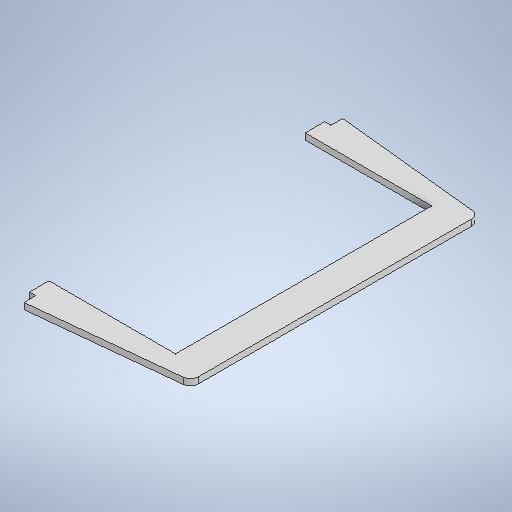
# Autodesk Inventor part: horazontal battery suport
Saved by Autodesk Inventor 2025.2 (Build 292293000, 293)
## iProperties
Created: 2025-01-25
Part Number: horazontal battery suport
Material: Generic
Document SubType Name: Modeling
Designer: alex
Density: 1 g/cm^3
Appearance: Default
Author: alex
Autodesk Inventor part; units mm, degrees
ref_plane "YZ Plane" through (0, 0, 0) normal (1, 0, 0) x (0, 1, 0)
ref_plane "XZ Plane" through (0, 0, 0) normal (0, 1, 0) x (-1, 0, 0)
ref_plane "XY Plane" through (0, 0, 0) normal (0, 0, 1) x (1, 0, 0)
sketch "Sketch1" plane through (0, 0, 0) normal (0, 1, 0) x (-1, 0, 0)
  line L0 (0, 0) -> (0, 31.75)
  line L1 (0, 31.75) -> (-10.16, 31.75)
  line L2 (-10.16, 31.75) -> (-10.16, 50.8)
  line L3 (-256.504, 13.9421) -> (-256.504, -430.5021)
  line L4 (-10.16, -467.36) -> (-10.16, -448.31)
  line L5 (-10.16, -448.31) -> (0, -448.31)
  line L6 (0, -448.31) -> (0, -416.56)
  line L7 (0, 0) -> (-205.704, 0)
  line L8 (-205.704, 0) -> (-205.704, -416.56)
  line L9 (-205.704, -416.56) -> (0, -416.56)
  line L10 (-245.1066, -443.1352) -> (-10.16, -467.36)
  line L11 (-245.1066, 26.5752) -> (-10.16, 50.8)
  arc A0 (-245.1066, 26.5752) -> (-256.504, 13.9421) centre (-243.804, 13.9421) ccw
  arc A1 (-256.504, -430.5021) -> (-245.1066, -443.1352) centre (-243.804, -430.5021) ccw
  point P0 (-256.504, 25.4)
  point P1 (-256.504, -441.96)
  dimension "d0" = 31.75
  dimension "d1" = 19.05
  dimension "d2" = 247.65
  dimension "d4" = 19.05
  dimension "d5" = 31.75
  dimension "d6" = 50.8
  dimension "d7" = 10.16
  dimension "d8" = 247.65
  dimension "d9" = 10.16
  dimension "d10" = 25.4
  dimension "d11" = 25.4
  dimension "d12" = 12.7
  constraints: 24 end point, 6 perpendicular, 4 point on circle, 4 point on line, 4 tangent, 2 centre point, 1 equal radius, 1 horizontal, 1 vertical
  measures "d0" distance of L0.start L0.end
  measures "d1" distance of L1.end L2.end
  measures "d2" distance of L2.end point (-256.504, 25.4)
  measures "d4" distance of L4.start L4.end
  measures "d5" distance of L5.end L6.end
  measures "d6" distance between parallel lines of L3 L8
  measures "d7" distance between parallel lines of L4 L6
  measures "d8" distance of point (-256.504, -441.96) L4.start
  measures "d9" distance of L0.end L1.end
  measures "d10" vertical distance of L8.end point (-256.504, -441.96)
  measures "d11" vertical distance of L7.end point (-256.504, 25.4)
  measures "d12" radius of A0
extrude "Extrusion1" add sketch "Sketch1" along normal blind 10.16
body "Solid1"
